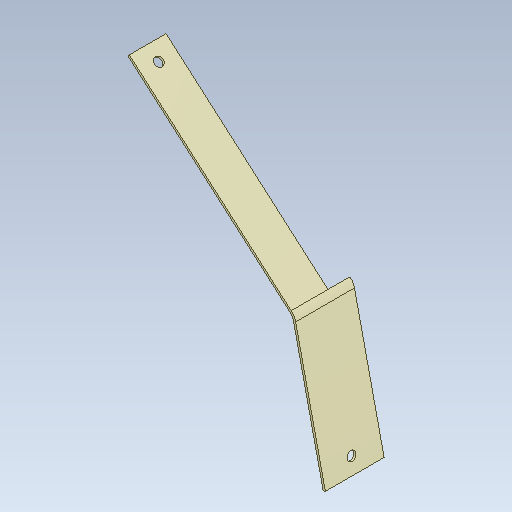
# Autodesk Inventor part: アームガードfull
Saved by Autodesk Inventor 2020.2 (Build 242310000, 310)
## iProperties
Created: 2020-03-30
Part Number: アームガードfull
Material: ポリプロピレン
Document SubType Name: Modeling
Designer: aoyama
Density: 0.899 g/cm^3
Appearance: 滑らか - 灰色
Author: aoyama
Autodesk Inventor part; units mm, degrees
ref_plane "YZ Plane" through (0, 0, 0) normal (1, 0, 0) x (0, 1, 0)
ref_plane "XZ Plane" through (0, 0, 0) normal (0, 1, 0) x (-1, 0, 0)
ref_plane "XY Plane" through (0, 0, 0) normal (0, 0, 1) x (1, 0, 0)
sketch "スケッチ1" plane through (0, 0, 0) normal (0, 0, 1) x (1, 0, 0)
  circle A0 centre (54.6996, 44) radius 4
  line L0 (62.6996, 0) -> (65.6996, 0)
  circle A1 centre (-0.366, 91.8281) radius 4
  circle A2 centre (-0.366, 91.8281) radius 4
  circle A3 centre (54.6996, 44) radius 4
  line L1 (58.602, 44.878) -> (68.6996, 0)
  line L2 (2.257, 94.8481) -> (57.3226, 47.0199)
  line L3 (2.7488, 95.4143) -> (57.8144, 47.5861)
  line L4 (59.3337, 45.0427) -> (69.4313, 0.1646)
  circle A4 centre (54.6996, 44) radius 4.75
  line L5 (2.257, 94.8481) -> (2.7488, 95.4143)
  line L6 (68.6996, 0) -> (69.4313, 0.1646)
  point P0 (0, 0)
  dimension "d0" = 0.75
  dimension "d1" = 0.75
  dimension "d2" = 0.75
  constraints: 14 end point, 2 centre point, 2 parallel, 2 perpendicular, 1 horizontal, 21 other
  measures "d0" distance between parallel lines of L2 L3
  measures "d1" distance between parallel lines of L1 L4
extrude "押し出し1" add sketch "スケッチ1" along normal blind 20 contours A0 L2 A4 L1 | A4 L4 L6 L1 | L2 L5 L3 A4 picked at (56.3248, 48.0683)
sketch "スケッチ2" plane through (2.7488, 95.4143, 20) normal (0.6557, 0.755, 0) x (0.755, -0.6557, 0)
  line L0 (72.9366, 20) -> (0, 20) projected
  line L1 (0, 20) -> (0, 0) projected
  line L2 (72.9366, 0) -> (0, 0) projected
  line L3 (72.9366, 20) -> (72.9366, 0) projected
  line L4 (5, 0) -> (5, 20)
  circle A0 centre (5, 6.25) radius 1.5
  line L5 (72.9366, 12.5) -> (0, 12.5)
  point P0 (60.4926, 20)
  dimension "d5" = 5
  dimension "d6" = 3
  dimension "d7" = 6.25
  dimension "d15" = 7.5
  constraints: 5 point on line, 4 end point, 1 centre point
  measures "d5" distance between parallel lines of L1 L4
  measures "d6" diameter of A0
  measures "d7" distance from line of L2 A0.centre
  measures "d15" distance between parallel lines of L0 L5
sketch "スケッチ3" plane through (59.3337, 45.0427, 20) normal (0.9756, 0.2195, 0) x (0, 0, -1)
  line L0 (20, -46) -> (20, 0) projected
  line L1 (20, 0) -> (0, 0) projected
  line L2 (0, -46) -> (0, 0) projected
  line L3 (20, -46) -> (0, -46) projected
  line L4 (0, -41) -> (20, -41)
  circle A0 centre (10, -41) radius 1.5
  point P0 (20, -30.9196)
  dimension "d8" = 5
  dimension "d9" = 3
  dimension "d10" = 10
  constraints: 2 end point, 2 point on line, 1 centre point, 1 horizontal, 1 midpoint
  measures "d8" distance between parallel lines of L4 L3
  measures "d9" diameter of A0
  measures "d10" distance from line of L0 A0.centre
extrude "押し出し2" cut sketch "スケッチ2" against normal blind 10 contours L3 L5 L4 L0 | L4 L5 L1 L0 | A0 L4 | L4 A0
extrude "押し出し3" cut sketch "スケッチ3" against normal blind 10 contours A0 L4 | L4 A0
